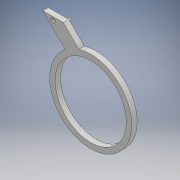
# Autodesk Inventor part: Float Walls
Saved by Autodesk Inventor 2017 (Build 210142000, 142)
## iProperties
Created: 2017-05-28
Part Number: Float Walls
Material: Generic
Document SubType Name: Modeling
Designer: William
Density: 1 g/cm^3
Appearance: Default
Author: William
Autodesk Inventor part; units mm, degrees
ref_plane "YZ Plane" through (0, 0, 0) normal (1, 0, 0) x (0, 1, 0)
ref_plane "XZ Plane" through (0, 0, 0) normal (0, 1, 0) x (-1, 0, 0)
ref_plane "XY Plane" through (0, 0, 0) normal (0, 0, 1) x (1, 0, 0)
sketch "Sketch1" plane through (0, 0, 0) normal (0, 1, 0) x (-1, 0, 0)
  line L0 (0, 0) -> (15, 0)
  circle A0 centre (7.5, -2.5) radius 1.6
  line L1 (15, 0) -> (44.3967, 0) construction
  line L2 (0, 0) -> (21.2132, 0) construction
  circle A1 centre (-20, -40) radius 26
  arc A2 (-11.2917, -11.2917) -> (-1.4346, -16.4346) centre (-20, -40) ccw
  line L3 (15, 0) -> (-1.4346, -16.4346)
  line L4 (0, 0) -> (-11.2917, -11.2917)
  line L5 (0, 0) -> (15.9689, 0) construction
  dimension "d0" = 15
  dimension "d1" = 2.5
  dimension "d2" = 7.5
  dimension "d3" = 3.2
  dimension "d6" = 52
  dimension "d7" = 40
  dimension "d8" = 60
  dimension "d10" = 20
  dimension "d11" = 135
  constraints: 12 end point, 4 horizontal, 3 centre point, 2 point on circle, 1 coincident, 1 equal length
  measures "d0" distance of L0.start L0.end
  measures "d1" distance from line of L0 A0.centre
  measures "d2" horizontal distance of L0.end A0.centre
  measures "d3" diameter of A0
  measures "d6" diameter of A1
  measures "d7" vertical distance of L0.start A1.centre
  measures "d8" diameter of A2
  measures "d10" horizontal distance of L0.start A1.centre
  measures "d11" angle of L4 L5
extrude "Extrusion1" add sketch "Sketch1" along normal blind 4
sketch "Sketch2" plane through (0, 4, 0) normal (0, 1, 0) x (1, 0, 0)
  point P0 (0, 0)
body "Solid1"
